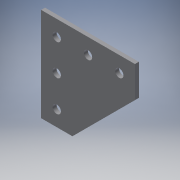
# Autodesk Inventor part: gusset
Saved by Autodesk Inventor 2016 (Build 200138000, 138)
## iProperties
Created: 2016-04-20
Part Number: gusset
Material: Generic
Document SubType Name: Modeling
Designer: gus
Density: 1 g/cm^3
Appearance: Default
Author: gus
Autodesk Inventor part; units mm, degrees
ref_plane "YZ Plane" through (0, 0, 0) normal (1, 0, 0) x (0, 1, 0)
ref_plane "XZ Plane" through (0, 0, 0) normal (0, 1, 0) x (-1, 0, 0)
ref_plane "XY Plane" through (0, 0, 0) normal (0, 0, 1) x (1, 0, 0)
sketch "Sketch1" plane through (0, 0, 0) normal (0, 0, 1) x (1, 0, 0)
  line L0 (0, 0) -> (0, -76.2)
  line L1 (0, -76.2) -> (25.4, -76.2)
  line L2 (25.4, -76.2) -> (76.2, -25.4)
  line L3 (76.2, -25.4) -> (76.2, 0)
  line L4 (76.2, 0) -> (0, 0)
  line L5 (12.7, -76.2) -> (12.7, 0) construction
  line L6 (0, -12.7) -> (76.2, -12.7) construction
  circle A0 centre (12.7, -12.7) radius 3.3734
  circle A1 centre (12.7, -38.1) radius 3.3734
  circle A2 centre (12.7, -63.5) radius 3.3734
  circle A3 centre (38.1, -12.7) radius 3.3734
  circle A4 centre (63.5, -12.7) radius 3.3734
  dimension "d0" = 76.2
  dimension "d1" = 25.4
  dimension "d2" = 12.7
  dimension "d3" = 6.7469
  dimension "d4" = 6.7469
  dimension "d5" = 6.7469
  dimension "d6" = 6.7469
  dimension "d7" = 6.7469
  dimension "d8" = 63.5
  dimension "d9" = 25.4
  dimension "d10" = 25.4
  dimension "d11" = 25.4
  constraints: 14 end point, 6 point on line, 5 centre point, 5 perpendicular, 4 midpoint, 1 parallel, 1 vertical
  measures "d0" distance of L0.start L0.end
  measures "d1" distance of L0.end L1.end
  measures "d2" distance of L0.start L6.start
  measures "d3" diameter of A0
  measures "d4" diameter of A1
  measures "d5" diameter of A2
  measures "d6" diameter of A3
  measures "d7" diameter of A4
  measures "d8" distance from line of L0 A4.centre
  measures "d9" distance of A3.centre A0.centre
  measures "d10" distance of A1.centre A0.centre
  measures "d11" distance of A2.centre A1.centre
extrude "Extrusion1" add sketch "Sketch1" along normal blind 3.175
body "Solid1"
